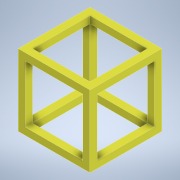
# Autodesk Inventor part: CUBE for Game Design_2
Saved by Autodesk Inventor 2021 (Build 250183000, 183)
## iProperties
Created: 2021-01-26
Part Number: CUBE for Game Design_2
Material: Generic
Document SubType Name: Modeling
Designer: aidan
Density: 1 g/cm^3
Appearance: Default
Author: aidan
Autodesk Inventor part; units mm, degrees
ref_plane "YZ Plane" through (0, 0, 0) normal (1, 0, 0) x (0, 1, 0)
ref_plane "XZ Plane" through (0, 0, 0) normal (0, 1, 0) x (-1, 0, 0)
ref_plane "XY Plane" through (0, 0, 0) normal (0, 0, 1) x (1, 0, 0)
sketch "Sketch1" plane through (0, 0, 0) normal (0, 0, 1) x (1, 0, 0)
  line L0 (0, 0) -> (254, 0)
  line L1 (254, 0) -> (254, 254)
  line L2 (254, 254) -> (0, 254)
  line L3 (0, 254) -> (0, 0)
  line L4 (25.4, 228.6) -> (228.6, 228.6)
  line L5 (228.6, 228.6) -> (228.6, 25.4)
  line L6 (228.6, 25.4) -> (25.4, 25.4)
  line L7 (25.4, 25.4) -> (25.4, 228.6)
  dimension "d0" = 254
  dimension "d1" = 25.4
  constraints: 16 end point, 4 parallel, 3 perpendicular, 1 horizontal, 3 other
  measures "d0" distance of L1.end L2.end
  measures "d1" distance between parallel lines of L2 L4
extrude "Extrusion1" add sketch "Sketch1" along normal blind 254
sketch "Sketch2" plane through (0, 254, 0) normal (0, 1, 0) x (1, 0, 0)
  line L0 (254, 0) -> (0, 0) projected
  line L1 (0, 0) -> (0, -254) projected
  line L2 (254, -254) -> (0, -254) projected
  line L3 (254, 0) -> (254, -254) projected
  line L4 (25.4, -228.6) -> (25.4, -25.4)
  line L5 (25.4, -25.4) -> (228.6, -25.4)
  line L6 (228.6, -25.4) -> (228.6, -228.6)
  line L7 (228.6, -228.6) -> (25.4, -228.6)
  dimension "d4" = 25.4
  constraints: 8 end point, 3 other
  measures "d4" distance between parallel lines of L1 L4
extrude "Extrusion2" cut sketch "Sketch2" against normal blind 254 contours L4 L5 L6 L7
sketch "Sketch3" plane through (254, 0, 0) normal (1, 0, 0) x (0, 0, -1)
  line L0 (0, 0) -> (0, 254) projected
  line L1 (0, 254) -> (-254, 254) projected
  line L2 (-254, 0) -> (-254, 254) projected
  line L3 (0, 0) -> (-254, 0) projected
  line L4 (0, 0) -> (0, 254) projected
  line L5 (-25.4, 228.6) -> (-25.4, 25.4)
  line L6 (-25.4, 25.4) -> (-228.6, 25.4)
  line L7 (-228.6, 25.4) -> (-228.6, 228.6)
  line L8 (-228.6, 228.6) -> (-25.4, 228.6)
  dimension "d7" = 25.4
  constraints: 8 end point, 3 other
  measures "d7" distance between parallel lines of L0 L5
extrude "Extrusion3" cut sketch "Sketch3" against normal blind 254 contours L5 L6 L7 L8
body "Solid1"
